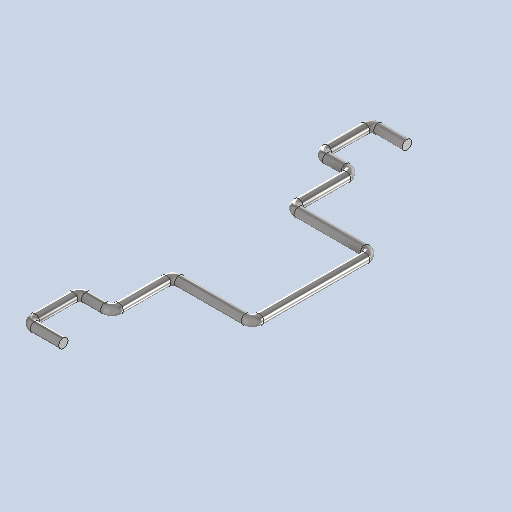
# Autodesk Inventor part: SeilspannerDraht
Saved by Autodesk Inventor 2025 (Build 290162010, 162A)
## iProperties
Created: 2024-11-27
Part Number: SeilspannerDraht
Material: Stahl, Kohlenstoff, Federstahl
Document SubType Name: Modeling
Designer: Admin
Density: 7.85 g/cm^3
Appearance: Halbpoliert(1)
Author: Admin
Autodesk Inventor part; units mm, degrees
ref_plane "YZ Plane" through (0, 0, 0) normal (1, 0, 0) x (0, 1, 0)
ref_plane "XZ Plane" through (0, 0, 0) normal (0, 1, 0) x (-1, 0, 0)
ref_plane "XY Plane" through (0, 0, 0) normal (0, 0, 1) x (1, 0, 0)
sketch "Skizze1" plane through (0, 0, 0) normal (0, 0, 1) x (1, 0, 0)
  line L0 (0, 0) -> (-3, 0)
  arc A0 (-3.7071, 0.7071) -> (-3, 0) centre (-3, 0.7071) ccw
  line L1 (-3, 0) -> (-3.7071, 0.7071) construction
  line L2 (-3, 0) -> (-2, 0) construction
  line L3 (-3.7071, 0.7071) -> (-3.7071, 4.7071)
  arc A1 (-1, 5.4142) -> (-0.2929, 6.1213) centre (-1, 6.1213) ccw
  line L4 (-0.2929, 6.1213) -> (-0.2929, 11.1213)
  arc A2 (0.4142, 11.8284) -> (-0.2929, 11.1213) centre (0.4142, 11.1213) ccw
  line L5 (-0.2929, 11.1213) -> (0.4142, 11.8284) construction
  line L6 (-0.2929, 11.1213) -> (0.7071, 11.1213) construction
  line L7 (0.4142, 11.8284) -> (7.4142, 11.8284)
  arc A3 (7.4142, 11.8284) -> (8.1213, 12.5355) centre (7.4142, 12.5355) ccw
  line L8 (7.4142, 11.8284) -> (8.1213, 12.5355) construction
  line L9 (7.4142, 11.8284) -> (8.4142, 11.8284) construction
  line L10 (8.1213, 12.5355) -> (8.1213, 18.1213)
  line L11 (8.1213, 18.1213) -> (-1.8787, 18.1213) construction
  line L12 (-1, 5.4142) -> (-3, 5.4142)
  arc A4 (-3, 5.4142) -> (-3.7071, 4.7071) centre (-3, 4.7071) ccw
  line L13 (0, 36.2426) -> (-3, 36.2426)
  arc A5 (-3, 36.2426) -> (-3.7071, 35.5355) centre (-3, 35.5355) ccw
  line L14 (-3, 36.2426) -> (-3.7071, 35.5355) construction
  line L15 (-3, 36.2426) -> (-2, 36.2426) construction
  line L16 (-3.7071, 35.5355) -> (-3.7071, 31.5355)
  arc A6 (-0.2929, 30.1213) -> (-1, 30.8284) centre (-1, 30.1213) ccw
  line L17 (-0.2929, 30.1213) -> (-0.2929, 25.1213)
  arc A7 (-0.2929, 25.1213) -> (0.4142, 24.4142) centre (0.4142, 25.1213) ccw
  line L18 (-0.2929, 25.1213) -> (0.4142, 24.4142) construction
  line L19 (-0.2929, 25.1213) -> (0.7071, 25.1213) construction
  line L20 (0.4142, 24.4142) -> (7.4142, 24.4142)
  arc A8 (8.1213, 23.7071) -> (7.4142, 24.4142) centre (7.4142, 23.7071) ccw
  line L21 (7.4142, 24.4142) -> (8.1213, 23.7071) construction
  line L22 (7.4142, 24.4142) -> (8.4142, 24.4142) construction
  line L23 (8.1213, 23.7071) -> (8.1213, 18.1213)
  line L24 (-1, 30.8284) -> (-3, 30.8284)
  arc A9 (-3.7071, 31.5355) -> (-3, 30.8284) centre (-3, 31.5355) ccw
  dimension "d0" = 3
  dimension "d1" = 1
  dimension "d2" = 135
  dimension "d5" = 1
  dimension "d6" = 5
  dimension "d7" = 1
  dimension "d8" = 45
  dimension "d9" = 7
  dimension "d10" = 1
  dimension "d11" = 45
  dimension "d12" = 4
  dimension "d16" = 6.1213
  dimension "d17" = 7
  dimension "d18" = 2
  dimension "d19" = 1
  dimension "d20" = 10
  constraints: 50 end point, 20 point on circle, 19 symmetric about line, 10 centre point, 10 tangent, 5 horizontal, 3 equal length, 1 coincident, 1 collinear, 1 vertical, 5 other
  measures "d0" distance of L0.start L0.end
  measures "d1" distance of L0.end L1.end
  measures "d2" angle of L2 L1
  measures "d5" distance of L12.start L4.start
  measures "d6" distance of L4.start L4.end
  measures "d7" distance of L4.end L5.end
  measures "d8" angle of L6 L5
  measures "d9" distance of L5.end L7.end
  measures "d10" distance of L7.end L8.end
  measures "d11" angle of L9 L8
  measures "d12" distance of L3.end L1.end
  measures "d16" vertical distance of L4.start L0.start
  measures "d17" distance from line of L10.end L6
  measures "d18" distance of L12.start L12.end
  measures "d19" distance of L12.end L3.end
  measures "d20" distance of L10.end L11.end
sketch "Skizze2" plane through (0, 0, 0) normal (1, 0, 0) x (0, 1, 0)
  circle A0 centre (0, 0) radius 0.5
  dimension "d21" = 1
  constraints: 1 centre point, 1 coincident
  measures "d21" diameter of A0
sweep "Sweeping1" add profiles "Skizze2" path "Skizze1"
